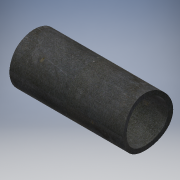
# Autodesk Inventor part: Nozzle 3 in
Saved by Autodesk Inventor 2016 (Build 200138000, 138)
## iProperties
Created: 2018-11-07
Part Number: Nozzle 3 in
Material: Steel ASTM A53 Gr.B
Document SubType Name: Modeling
Designer: Wijaya
Mass: 2956.55 g
Surface Area: 1064.05 cm^2
Volume: 390.046 cm^3
Density: 7.58 g/cm^3
Appearance: Semi-Polished
Author: Wijaya
Autodesk Inventor part; units mm, degrees
ref_plane "YZ Plane" through (0, 0, 0) normal (1, 0, 0) x (0, 1, 0)
ref_plane "XZ Plane" through (0, 0, 0) normal (0, 1, 0) x (-1, 0, 0)
ref_plane "XY Plane" through (0, 0, 0) normal (0, 0, 1) x (1, 0, 0)
sketch "Sketch4" plane through (0, 0, 0) normal (0, 0, 1) x (1, 0, 0)
  circle A0 centre (377.8, 0) radius 177.8
  point P0 (0, 0)
  dimension "d24" = 355.6
  dimension "d25" = 377.8
  constraints: 1 centre point, 1 horizontal alignment
  measures "d24" diameter of A0
  measures "d25" distance of point (0, 0) A0.centre
sketch "Sketch1" plane through (0, 0, 0) normal (0, 0, 1) x (1, 0, 0)
  line L0 (0, 0) -> (298.2609, 0)
  line L1 (0, 38.43) -> (4.6193, 44.45)
  line L2 (4.6193, 44.45) -> (205.6459, 44.45)
  line L3 (205.6459, 44.45) -> (205.6459, 36.83)
  line L4 (205.6459, 36.83) -> (0, 36.83)
  circle A0 centre (377.8, 0) radius 177.8 projected
  line L5 (0, 38.43) -> (0, 36.83)
  dimension "d2" = 73.66
  dimension "d3" = 88.9
  dimension "d4" = 1.6
  dimension "d29" = 37.5
  constraints: 12 end point, 2 perpendicular, 1 horizontal, 1 vertical alignment, 2 other
  measures "d2" diameter of L4 L0
  measures "d3" diameter of L2 L0
  measures "d4" distance from line of L4 L1.start
  measures "d29" angle of L5 L1
revolve "Revolution1" add sketch "Sketch1" angle 360 about axis through (0, 0, 0) along (1, 0, 0) picked at (205.4346, 41.0663) contours L1 L2 A0 L4 L5 | L3 L4 A0
extrude "Extrusion1" cut sketch "Sketch4" along normal mid plane 88.9
body "Solid1"
